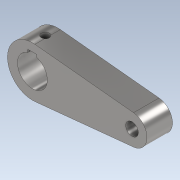
# Autodesk Inventor part: placa manivela
Saved by Autodesk Inventor 2021 (Build 250183000, 183)
## iProperties
Created: 2021-06-18
Part Number: placa manivela
Material: Steel, Carbon
Document SubType Name: Modeling
Designer: Andrés Holguín
Density: 7.85 g/cm^3
Appearance: Semi-Polished
Author: Andrés Holguín
Autodesk Inventor part; units mm, degrees
ref_plane "YZ Plane" through (0, 0, 0) normal (1, 0, 0) x (0, 1, 0)
ref_plane "XZ Plane" through (0, 0, 0) normal (0, 1, 0) x (-1, 0, 0)
ref_plane "XY Plane" through (0, 0, 0) normal (0, 0, 1) x (1, 0, 0)
sketch "Sketch1" plane through (0, 0, 0) normal (0, 1, 0) x (-1, 0, 0)
  arc A0 (9, -28.6182) -> (-9, -28.6182) centre (0, 0) ccw
  arc A1 (-5, 49.7494) -> (-5, -49.7494) centre (0, 0) ccw construction
  line L0 (0, 0) -> (-200, 0) construction
  arc A2 (-170, 0) -> (-200, 30) centre (-200, 0) ccw construction
  line L1 (-200, 30) -> (-200, -30) construction
  line L2 (-5, -49.7494) -> (-203, -29.8496)
  line L3 (-5, 49.7494) -> (-203, 29.8496)
  arc A3 (-5, -49.7494) -> (-5, 49.7494) centre (0, 0) ccw
  arc A4 (-200, -30) -> (-170, 0) centre (-200, 0) ccw construction
  arc A5 (-200, 30) -> (-200, -30) centre (-200, 0) ccw
  line L4 (0, 0) -> (0, -30) construction
  line L5 (9, -23) -> (-9, -23) construction
  line L6 (9, -23) -> (9, -28.6182) construction
  line L7 (-9, -23) -> (-9, -28.6182) construction
  line L8 (9, -28.6182) -> (9, -34)
  line L9 (-9, -28.6182) -> (-9, -34)
  line L10 (9, -34) -> (-9, -34)
  arc A6 (0, -30) -> (9, -28.6182) centre (0, 0) ccw construction
  arc A7 (-9, -28.6182) -> (0, -30) centre (0, 0) ccw construction
  dimension "d0" = 60
  dimension "d1" = 100
  dimension "d2" = 200
  dimension "d3" = 60
  dimension "d5" = 18
  dimension "d6" = 7
  dimension "d7" = 4
  constraints: 22 end point, 20 point on circle, 8 centre point, 6 tangent, 6 vertical, 3 coincident, 2 horizontal, 1 midpoint, 1 perpendicular, 1 point on line, 1 symmetric about line
  measures "d0" diameter of A0
  measures "d1" diameter of A1
  measures "d2" distance of L0.start L0.end
  measures "d3" diameter of A2
  measures "d5" distance of L5.start L5.end
  measures "d6" distance from line of L4.end L5
  measures "d7" distance from line of L10 L4.end
extrude "Extrusion1" add sketch "Sketch1" along normal blind 51.2
sketch "Sketch2" plane through (0, 51.2, 0) normal (0, 1, 0) x (1, 0, 0)
  arc A0 (203, -29.8496) -> (203, 29.8496) centre (200, 0) ccw projected
  circle A1 centre (200, 0) radius 12.7
  point P0 (0, 0)
  dimension "d10" = 25.4
  constraints: 1 centre point, 1 coincident
  measures "d10" diameter of A1
extrude "Extrusion4" cut sketch "Sketch2" against normal through all
sketch "Sketch4" plane through (-9, 0, -34) normal (0, 0, 1) x (1, 0, 0)
  line L0 (0, 0) -> (18, 0) projected
  line L1 (18, 0) -> (18, 51.2) projected
  line L2 (0, 51.2) -> (18, 51.2) projected
  line L3 (0, 0) -> (0, 51.2) projected
  line L4 (9, 51.2) -> (9, 0) construction
  line L5 (0, 0) -> (0, 51.2) construction
  line L6 (0, 25.6) -> (18, 25.6) construction
  circle A0 centre (9, 25.6) radius 7.9375
  dimension "d24" = 15.875
  constraints: 4 end point, 4 midpoint, 1 centre point, 1 vertical
  measures "d24" diameter of A0
extrude "Extrusion5" cut sketch "Sketch4" against normal through all contours A0
body "Solid1"
